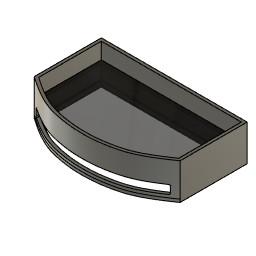
Hood v8 (Autodesk Fusion 360 design; units mm, degrees)
Autodesk Fusion 360 part; units mm, degrees
sketch "Core Shapes" plane through (0, 0, 0) normal (0, 0, 1) x (1, 0, 0) in component "Base"
  line L0 (-248.2316, 129.4806) -> (236.7684, 129.4806)
  line L1 (236.7684, 129.4806) -> (236.7684, -87.5194)
  line L2 (-248.2316, 129.4806) -> (-248.2316, -87.5194)
  line L3 (-248.2316, 129.5231) -> (-148.2316, 129.5231) construction
  line L4 (-148.2316, 129.5231) -> (-98.2316, 129.5231) construction
  line L5 (-98.2316, 129.5231) -> (-48.2316, 129.5231) construction
  line L6 (-48.2316, 129.5231) -> (-5.7316, 129.5231) construction
  line L7 (-5.7316, 129.5231) -> (36.7684, 129.5231) construction
  line L8 (36.7684, 129.5231) -> (86.7684, 129.5231) construction
  line L9 (86.7684, 129.5231) -> (136.7684, 129.5231) construction
  line L10 (136.7684, 129.5231) -> (236.7684, 129.5231) construction
  line L11 (-148.2316, 129.5231) -> (-198.2316, 129.5231) construction
  line L12 (136.7684, 129.5231) -> (186.7684, 129.5231) construction
  spline S0 degree 5 poles (236.7684, -87.5194) (233.1275, -90.0302) (225.9745, -94.9215) (215.632, -101.8683) (202.5885, -110.3609) (187.3699, -119.7584) (173.0488, -128.0191) (159.4416, -135.2303) (146.4596, -141.4515) (134.0705, -146.7334) (122.572, -151.0105) (111.8531, -154.404) (101.4383, -157.1926) (90.8478, -159.6546) (79.831, -161.9639) (68.6564, -164.0577) (57.4313, -165.9065) (46.2767, -167.4659) (35.2758, -168.7063) (24.5908, -169.5934) (14.2675, -170.1481) (4.2099, -170.4353) (-5.7316, -170.5197) (-15.6731, -170.4353) (-25.7306, -170.1481) (-36.054, -169.5934) (-46.739, -168.7063) (-57.7399, -167.4659) (-68.8945, -165.9065) (-80.1196, -164.0577) (-91.2942, -161.9639) (-102.311, -159.6546) (-112.9015, -157.1926) (-123.3162, -154.404) (-134.0352, -151.0105) (-145.5337, -146.7334) (-157.9227, -141.4515) (-170.9047, -135.2303) (-184.5119, -128.0191) (-198.833, -119.7584) (-214.0516, -110.3609) (-227.0952, -101.8683) (-237.4377, -94.9215) (-244.5906, -90.0302) (-248.2316, -87.5194) knots 0 0 0 0 0 0 0.025 0.05 0.075 0.1 0.125 0.15 0.175 0.2 0.225 0.25 0.275 0.3 0.325 0.35 0.375 0.4 0.425 0.45 0.475 0.5 0.525 0.55 0.575 0.6 0.625 0.65 0.675 0.7 0.725 0.75 0.775 0.8 0.825 0.85 0.875 0.9 0.925 0.95 0.975 1 1 1 1 1 1
  line L13 (-107.2415, -162.3529) -> (-189.2217, -128.601)
  line L14 (177.7585, -128.601) -> (95.7783, -162.3529)
  line L15 (135.0935, -150.2043) -> (38.4433, -170.7496)
  line L16 (87.2864, -163.3286) -> (-13.7495, -173.6253)
  line L17 (-194.6091, -124.4963) -> (-301.854, -50.5425)
  line L18 (-49.9065, -170.7496) -> (-146.5567, -150.2043)
  line L19 (42.7251, -170.4769) -> (-54.1883, -170.4769)
  line L20 (2.2864, -173.6253) -> (-98.7495, -163.3286)
  line L21 (290.3909, -50.5425) -> (183.146, -124.4963)
  line L22 (-243.2316, 124.4806) -> (-243.2316, -84.8908)
  spline S1 degree 3 poles (231.7684, -84.8908) (217.3788, -94.7744) (204.2713, -103.3892) (192.1696, -110.8472) (180.1437, -118.2584) (169.0625, -124.5455) (158.5798, -129.8924) (149.6167, -134.4641) (141.0669, -138.358) (133.067, -141.5863) (126.4355, -144.2624) (120.2487, -146.4561) (114.3178, -148.3059) (107.4423, -150.4504) (100.8301, -152.1666) (93.9436, -153.7637) (83.7713, -156.1229) (73.019, -158.2415) (62.3188, -160.001) (50.0743, -162.0144) (37.872, -163.5188) (26.3543, -164.3777) (15.113, -165.2159) (4.5057, -165.4844) (-6.1239, -165.4768) (-14.8447, -165.4705) (-23.5538, -165.2741) (-32.6324, -164.7271) (-40.7604, -164.2373) (-49.2319, -163.4407) (-57.9001, -162.3304) (-69.2622, -160.8751) (-80.9209, -158.9043) (-92.2733, -156.6066) (-98.3011, -155.3866) (-104.1945, -154.0922) (-109.9291, -152.6856) (-118.744, -150.5234) (-127.2665, -148.061) (-136.7487, -144.5845) (-146.7053, -140.9341) (-157.6972, -136.1597) (-169.3933, -130.2229) (-183.3807, -123.1231) (-198.4148, -114.3473) (-215.3707, -103.4548) (-224.109, -97.8413) (-233.3732, -91.6621) (-243.2316, -84.8908) knots 0.002992 0.002992 0.002992 0.002992 0.063009 0.063009 0.063009 0.122649 0.122649 0.122649 0.173644 0.173644 0.173644 0.215917 0.215917 0.215917 0.264922 0.264922 0.264922 0.33731 0.33731 0.33731 0.420147 0.420147 0.420147 0.500995 0.500995 0.500995 0.567324 0.567324 0.567324 0.626708 0.626708 0.626708 0.704547 0.704547 0.704547 0.745877 0.745877 0.745877 0.809408 0.809408 0.809408 0.876117 0.876117 0.876117 0.955895 0.955895 0.955895 0.997008 0.997008 0.997008 0.997008
  line L23 (231.7684, 124.4806) -> (231.7684, -84.8908)
  line L24 (-243.2316, 124.4806) -> (231.7684, 124.4806)
  line L25 (-258.2316, 139.4806) -> (-258.2316, -92.7707)
  spline S2 degree 3 poles (246.7684, -92.7707) (245.3274, -93.7644) (243.8864, -94.7581) (242.4453, -95.7518) (225.7569, -107.2598) (210.7047, -117.1426) (196.7986, -125.6013) (184.3271, -133.1874) (172.716, -139.6483) (161.651, -145.1386) (151.8202, -150.0164) (142.4121, -154.1302) (133.6456, -157.4724) (125.7623, -160.4778) (118.4348, -162.8441) (111.2999, -164.834) (104.1564, -166.8263) (97.1393, -168.4791) (89.8825, -170.0373) (76.5827, -172.8931) (62.696, -175.3451) (49.1114, -177.1097) (40.1096, -178.279) (31.2422, -179.1316) (22.7518, -179.6583) (12.6374, -180.2858) (3.0519, -180.4899) (-6.5222, -180.4764) (-14.9332, -180.4645) (-23.3749, -180.2792) (-32.2054, -179.7777) (-40.7828, -179.2905) (-49.751, -178.4758) (-58.8855, -177.3257) (-72.3312, -175.6329) (-86.101, -173.2519) (-99.348, -170.4621) (-106.0519, -169.0503) (-112.5575, -167.5587) (-119.0902, -165.8313) (-126.309, -163.9225) (-133.6234, -161.6908) (-141.4865, -158.8234) (-152.2718, -154.8905) (-164.0767, -149.7598) (-176.5488, -143.4124) (-189.4298, -136.8569) (-203.0426, -129.002) (-217.961, -119.5883) (-229.111, -112.5525) (-241.0276, -104.6342) (-253.9085, -95.7518) (-255.3495, -94.7581) (-256.7905, -93.7644) (-258.2316, -92.7707) knots -0.005937 -0.005937 -0.005937 -0.005937 0 0 0 0.06828 0.06828 0.06828 0.129516 0.129516 0.129516 0.183921 0.183921 0.183921 0.232844 0.232844 0.232844 0.281827 0.281827 0.281827 0.371598 0.371598 0.371598 0.431085 0.431085 0.431085 0.501951 0.501951 0.501951 0.564207 0.564207 0.564207 0.624678 0.624678 0.624678 0.713689 0.713689 0.713689 0.758734 0.758734 0.758734 0.808511 0.808511 0.808511 0.876786 0.876786 0.876786 0.947299 0.947299 0.947299 1 1 1 1.005937 1.005937 1.005937 1.005937
  line L26 (246.7684, 139.4806) -> (246.7684, -92.7707)
  line L27 (-258.2316, 139.4806) -> (246.7684, 139.4806)
  point P0 (136.7684, -145.4769)
  point P1 (86.7684, -160.4769)
  point P2 (36.7684, -168.4769)
  point P3 (-5.7316, -170.4769)
  point P4 (-98.2316, -160.4769)
  point P5 (-148.2316, -145.4769)
  dimension "d1" = 485
  dimension "d2" = 217
  dimension "d3" = 217
  dimension "d4" = 100
  dimension "d5" = 50
  dimension "d6" = 50
  dimension "d7" = 42.5
  dimension "d8" = 42.5
  dimension "d9" = 50
  dimension "d10" = 50
  dimension "d11" = 100
  dimension "d12" = 275
  dimension "d13" = 290
  dimension "d14" = 298
  dimension "d15" = 300
  dimension "d16" = 298
  dimension "d17" = 290
  dimension "d18" = 275
  dimension "d19" = 50
  dimension "d21" = 50
  constraint perpendicular L0 L1
  constraint perpendicular L0 L2
  constraint coincident L2 L3.start
  constraint perpendicular L2 L3
  constraint parallel L3 L4
  constraint parallel L4 L5
  constraint parallel L0 L6
  constraint parallel L0 L7
  constraint parallel L0 L8
  constraint parallel L0 L9
  constraint parallel L0 L10
  constraint midpoint P5 L13
  constraint midpoint P0 L14
  constraint midpoint P1 L15
  constraint midpoint P2 L16
  constraint midpoint L2.end L17
  constraint midpoint P4 L18
  constraint midpoint P3 L19
  constraint midpoint L1.end L21
  constraint parallel L2 L22
  constraint parallel L1 L23
  constraint parallel L0 L24
  constraint parallel L2 L25
  constraint parallel L1 L26
  constraint parallel L0 L27
  measures "d1" distance of L0.start L0.end
  measures "d2" distance of L0.end L1.end
  measures "d3" distance of L0.start L2.end
  measures "d4" distance of L3.start L3.end
  measures "d5" distance of L3.end L4.end
  measures "d6" distance of L4.end L5.end
  measures "d7" distance of L5.end L6.end
  measures "d8" distance of L6.end L7.end
  measures "d9" distance of L7.end L8.end
  measures "d10" distance of L8.end L9.end
  measures "d11" distance of L9.end L10.end
  measures "d12" distance of L9.end P0
  measures "d13" distance of L8.end P1
  measures "d14" distance of L7.end P2
  measures "d15" distance of L6.end P3
  measures "d17" distance of L4.end P4
  measures "d18" distance of L3.end P5
  measures "d19" distance of L3.end L11.end
  measures "d21" distance of L9.end L12.end
extrude "Extrude4" add sketch "Core Shapes" against normal blind 7 contours L0 L1 L2 S0 makes body 1 in component "Base"
extrude "Extrude5" add sketch "Core Shapes" along normal blind 10 bodies 1 in component "Base"
extrude "Extrude6" add sketch "Core Shapes" along normal blind 50 from surface at 10 contours L0 L1 L2 L17 L21 L25 L26 L27 | S0 L13 L14 L15 L16 L17 L18 L19 L20 L21 L25 S2 L26 | S0 L13 L18 | S0 L14 L15 | S0 L18 L20 | S0 L15 L16 | S0 L19 L20 | L18 L19 L20 | S0 L16 L19 | L15 L16 L19 | L16 L19 L20 bodies 1 in component "Base"
extrude "Extrude7" add sketch "Core Shapes" along normal blind 5 from surface at 60 bodies 1 in component "Base"
extrude "Extrude8" add sketch "Core Shapes" along normal blind 60 from surface at 65 contours L0 L1 L2 L17 L21 L25 L26 L27 | S0 L13 L14 L15 L16 L17 L18 L19 L20 L21 L25 S2 L26 | S0 L13 L18 | S0 L14 L15 | S0 L18 L20 | S0 L15 L16 | S0 L19 L20 | L18 L19 L20 | S0 L16 L19 | L15 L16 L19 | L16 L19 L20 bodies 1 in component "Base"
sketch "Ventilation" plane through (0, 129.4806, 0) normal (0, -1, 0) x (1, 0, 0)
  line L0 (-248.2316, 10) -> (236.7684, 10) construction
  line L1 (236.7684, 10) -> (236.7684, 60) construction
  line L2 (236.7684, 60) -> (-248.2316, 60) construction
  line L3 (-248.2316, 60) -> (-248.2316, 10) construction
  line L4 (-248.2316, 60) -> (236.7684, 60) construction
  line L5 (236.7684, 60) -> (236.7684, 10) construction
  line L6 (236.7684, 10) -> (-248.2316, 10) construction
  line L7 (-248.2316, 10) -> (-248.2316, 60) construction
  line L8 (223.7684, 20) -> (-235.2316, 20)
  line L9 (-238.2316, 23) -> (-238.2316, 47)
  line L10 (-235.2316, 50) -> (223.7684, 50)
  line L11 (226.7684, 47) -> (226.7684, 23)
  arc A0 (-235.2316, 50) -> (-238.2316, 47) centre (-235.2316, 47) ccw
  arc A1 (226.7684, 47) -> (223.7684, 50) centre (223.7684, 47) ccw
  arc A2 (223.7684, 20) -> (226.7684, 23) centre (223.7684, 23) ccw
  arc A3 (-238.2316, 23) -> (-235.2316, 20) centre (-235.2316, 23) ccw
  dimension "d48" = 3
  dimension "d49" = 3
  dimension "d50" = 3
  dimension "d51" = 3
  constraint horizontal L4
  constraint vertical L5
  constraint horizontal L6
  constraint vertical L7
  constraint coincident L0.end L1.start
  constraint coincident L2.end L3.start
  constraint parallel L6 L8
  constraint parallel L7 L9
  constraint parallel L4 L10
  constraint parallel L5 L11
  constraint tangent L9 A0
  constraint tangent L10 A0
  constraint tangent L11 A1
  constraint tangent L10 A1
  constraint tangent L11 A2
  constraint tangent L8 A2
  constraint tangent L8 A3
  constraint tangent L9 A3
  measures "d48" radius of A0
  measures "d49" radius of A1
  measures "d50" radius of A2
  measures "d51" radius of A3
extrude "Extrude1" add sketch "Core Shapes" along normal blind 4 from surface at 65 separate body contours L0 L1 L2 S0 | L22 S1 L23 L24 makes body 2
extrude "Extrude9" cut sketch "Ventilation" along normal blind 370 bodies 1 in component "Base"
component "Base" placed x (1, 0, 0) y (0, 1, 0) z (0, 0, 1) at (0, 0, 0)
named bodies: "Glass"
